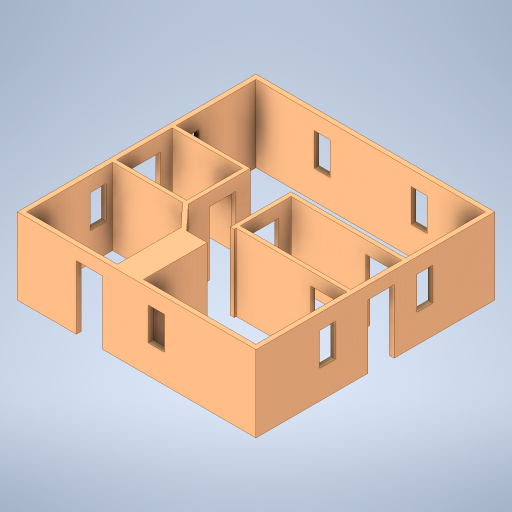
# Autodesk Inventor part: Existing_Kitchen_And_Dining_Room
Saved by Autodesk Inventor 2024 (Build 280153000, 153)
## iProperties
Created: 2023-04-15
Part Number: Existing_Kitchen_And_Dining_Room
Material: Generic
Document SubType Name: Modeling
Designer: Tom
Density: 1 g/cm^3
Appearance: Cherry - Natural Low Gloss
Author: Tom
Autodesk Inventor part; units mm, degrees
ref_plane "YZ Plane" through (0, 0, 0) normal (1, 0, 0) x (0, 1, 0)
ref_plane "XZ Plane" through (0, 0, 0) normal (0, 1, 0) x (-1, 0, 0)
ref_plane "XY Plane" through (0, 0, 0) normal (0, 0, 1) x (1, 0, 0)
sketch "Sketch1" plane through (0, 0, 0) normal (0, 1, 0) x (-1, 0, 0)
  line L0 (149.225, -7470.775) -> (149.225, 149.225)
  line L1 (149.225, 149.225) -> (-7470.775, 149.225)
  line L2 (-7470.775, 149.225) -> (-7470.775, -7470.775)
  line L3 (-7470.775, -7470.775) -> (149.225, -7470.775)
  line L4 (149.225, -2876.55) -> (149.225, -3028.95)
  line L5 (0, 0) -> (0, -7321.55)
  line L6 (0, -7321.55) -> (-7321.55, -7321.55)
  line L7 (-7321.55, -7321.55) -> (-7321.55, 0)
  line L8 (-7321.55, 0) -> (0, 0)
  line L9 (0, -2743.2) -> (-2235.2, -2743.2)
  line L10 (-2235.2, -2743.2) -> (-2895.6, -2032)
  line L11 (-2895.6, -2032) -> (-2895.6, 0)
  line L12 (0, -2873.375) -> (-2235.2, -2873.375)
  line L13 (-2235.2, -2873.375) -> (-2235.2, -4645.3435)
  line L14 (-2235.2, -4645.3435) -> (0, -4645.3435)
  line L15 (0, -4775.5185) -> (-2365.375, -4775.5185)
  line L16 (-2365.375, -4775.5185) -> (-2365.375, -2794.3185)
  line L17 (-2365.375, -2794.3185) -> (-3073.2421, -2032)
  line L18 (-3073.2421, -2032) -> (-3733.6421, -2032)
  line L19 (-3733.6421, -2032) -> (-3733.6421, 0)
  line L20 (-7321.55, -3025.775) -> (-3794.125, -3025.775)
  line L21 (-3794.125, -3025.775) -> (-3794.125, -4645.3435)
  line L22 (-3663.95, -4775.5185) -> (-3663.95, -2832.1)
  line L23 (-3794.125, -2895.6) -> (-7321.55, -2895.6)
  line L24 (-3663.95, -4775.5185) -> (-7321.55, -4775.5185)
  line L25 (-7321.55, -4645.3435) -> (-3794.125, -4645.3435)
  line L26 (-3794.125, -2895.6) -> (-3794.125, -2832.1)
  line L27 (-3794.125, -2832.1) -> (-3663.95, -2832.1)
  dimension "d34" = 7620
  dimension "d37" = 149.225
  dimension "d38" = 7620
  dimension "d39" = 2743.2
  dimension "d40" = 2032
  dimension "d42" = 2235.2
  dimension "d44" = 130.175
  dimension "d47" = 130.175
  dimension "d48" = 1981.2
  dimension "d49" = 130.175
  dimension "d50" = 130.175
  dimension "d52" = 2032
  dimension "d53" = 2895.6
  dimension "d57" = 2895.6
  dimension "d58" = 130.175
  dimension "d62" = 660.4
  dimension "d142" = 130.175
  dimension "d143" = 63.5
  dimension "d144" = 3657.6
  constraints: 56 end point, 12 perpendicular, 10 point on line, 6 horizontal, 4 collinear, 3 parallel, 1 coincident, 3 other
  measures "d34" distance of L1.end L2.end
  measures "d37" distance between parallel lines of L0 L5
  measures "d38" distance of L2.end L0.start
  measures "d39" distance between parallel lines of L8 L9
  measures "d40" distance of L10.end L11.end
  measures "d42" distance of L12.start L12.end
  measures "d44" distance between parallel lines of L9 L12
  measures "d47" distance between parallel lines of L13 L16
  measures "d48" distance of L15.end L16.end
  measures "d49" distance between parallel lines of L15 L14
  measures "d50" distance between parallel lines of L10 L17
  measures "d52" distance of L18.end L19.end
  measures "d53" distance between parallel lines of L5 L11
  measures "d57" distance between parallel lines of L8 L23
  measures "d58" distance between parallel lines of L20 L23
  measures "d62" distance of L17.end L18.end
  measures "d142" distance between parallel lines of L21 L22
  measures "d143" distance between parallel lines of L27 L23
  measures "d144" distance between parallel lines of L7 L22
extrude "Extrusion1" add sketch "Sketch1" along normal blind 2438.4 contours L3 L2 L1 L0 | L5 L12 L13 L14 L15 L16 L17 L18 L19 L8 L11 L10 L9 | L23 L26 L27 L22 L24 L7 L25 L21 L20
sketch "Sketch2" plane through (-149.225, 0, -7470.775) normal (-1, 0, 0) x (0, 0, 1)
  line L0 (4937.125, 1955.8) -> (5445.125, 1955.8)
  line L1 (5445.125, 1955.8) -> (5445.125, 914.4)
  line L2 (5445.125, 914.4) -> (4937.125, 914.4)
  line L3 (4937.125, 914.4) -> (4937.125, 1955.8)
  line L4 (0, 0) -> (7620, 0) projected
  line L5 (2485.7065, 1955.8) -> (1977.7065, 1955.8)
  line L6 (1977.7065, 1955.8) -> (1977.7065, 914.4)
  line L7 (1977.7065, 914.4) -> (2485.7065, 914.4)
  line L8 (2485.7065, 914.4) -> (2485.7065, 1955.8)
  line L9 (3193.7315, 1955.8) -> (4235.1315, 1955.8)
  line L10 (4235.1315, 1955.8) -> (4235.1315, 914.4)
  line L11 (4235.1315, 914.4) -> (3193.7315, 914.4)
  line L12 (3193.7315, 914.4) -> (3193.7315, 1955.8)
  point P0 (7470.775, 0)
  point P1 (4727.575, 2438.4)
  point P2 (2695.2565, 2438.4)
  point P3 (2825.4315, 2438.4)
  dimension "d63" = 914.4
  dimension "d64" = 209.55
  dimension "d65" = 508
  dimension "d66" = 1041.4
  dimension "d67" = 209.55
  dimension "d68" = 508
  dimension "d69" = 1041.4
  dimension "d70" = 914.4
  dimension "d71" = 914.4
  dimension "d72" = 1041.4
  dimension "d73" = 1041.4
  dimension "d74" = 368.3
  constraints: 24 end point, 6 parallel, 3 horizontal, 3 perpendicular
  measures "d63" distance between parallel lines of L4 L2
  measures "d64" distance from line of L3 point (4727.575, 2438.4)
  measures "d65" distance of L0.start L0.end
  measures "d66" distance of L0.end L1.end
  measures "d67" distance from line of L8 point (2695.257, 2438.4)
  measures "d68" distance of L5.start L5.end
  measures "d69" distance of L5.end L6.end
  measures "d70" distance between parallel lines of L4 L7
  measures "d71" distance between parallel lines of L4 L11
  measures "d72" distance of L11.end L9.start
  measures "d73" distance of L9.start L9.end
  measures "d74" distance from line of L12 point (2825.432, 2438.4)
extrude "Extrusion2" cut sketch "Sketch2" against normal up to surface (149.225 mm away)
sketch "Sketch3" plane through (7470.775, 0, -7470.775) normal (0, 0, -1) x (-1, 0, 0)
  line L0 (5105.4, 1955.8) -> (5613.4, 1955.8)
  line L1 (5613.4, 1955.8) -> (5613.4, 914.4)
  line L2 (5613.4, 914.4) -> (5105.4, 914.4)
  line L3 (5105.4, 914.4) -> (5105.4, 1955.8)
  line L4 (0, 0) -> (7620, 0) projected
  line L5 (7470.775, 0) -> (7470.775, 2438.4) projected
  line L6 (2006.6, 1955.8) -> (2514.6, 1955.8)
  line L7 (2514.6, 1955.8) -> (2514.6, 914.4)
  line L8 (2514.6, 914.4) -> (2006.6, 914.4)
  line L9 (2006.6, 914.4) -> (2006.6, 1955.8)
  line L10 (149.225, 0) -> (149.225, 2438.4) projected
  dimension "d78" = 1041.4
  dimension "d79" = 508
  dimension "d80" = 2365.375
  dimension "d81" = 2365.375
  dimension "d82" = 1041.4
  dimension "d83" = 508
  dimension "d84" = 914.4
  dimension "d85" = 914.4
  constraints: 16 end point, 4 parallel, 2 horizontal, 2 perpendicular
  measures "d78" distance of L0.end L1.end
  measures "d79" distance of L0.start L0.end
  measures "d80" distance between parallel lines of L5 L3
  measures "d81" distance between parallel lines of L10 L7
  measures "d82" distance of L6.end L7.end
  measures "d83" distance of L6.start L6.end
  measures "d84" distance between parallel lines of L4 L8
  measures "d85" distance between parallel lines of L4 L2
extrude "Extrusion3" cut sketch "Sketch3" against normal up to surface (149.225 mm away)
sketch "Sketch4" plane through (7470.775, 0, 149.225) normal (1, 0, 0) x (0, 0, -1)
  line L0 (5134.2935, 1955.8) -> (5642.2935, 1955.8)
  line L1 (5642.2935, 1955.8) -> (5642.2935, 914.4)
  line L2 (5642.2935, 914.4) -> (5134.2935, 914.4)
  line L3 (5134.2935, 914.4) -> (5134.2935, 1955.8)
  line L4 (0, 0) -> (7620, 0) projected
  line L5 (2533.65, 1955.8) -> (2025.65, 1955.8)
  line L6 (2025.65, 1955.8) -> (2025.65, 914.4)
  line L7 (2025.65, 914.4) -> (2533.65, 914.4)
  line L8 (2533.65, 914.4) -> (2533.65, 1955.8)
  line L9 (0, 0) -> (0, 2438.4) projected
  line L10 (4794.5685, 0) -> (3175, 0) projected
  line L11 (4410.2347, 0) -> (3572.0347, 0)
  line L12 (3572.0347, 0) -> (3572.0347, 2032)
  line L13 (3572.0347, 2032) -> (4410.2347, 2032)
  line L14 (4410.2347, 2032) -> (4410.2347, 0)
  point P0 (149.225, 0)
  point P1 (4924.7435, 2438.4)
  point P2 (4794.5685, 2438.4)
  dimension "d88" = 209.55
  dimension "d89" = 508
  dimension "d90" = 1041.4
  dimension "d91" = 914.4
  dimension "d92" = 508
  dimension "d94" = 1041.4
  dimension "d97" = 2533.65
  dimension "d98" = 914.4
  dimension "d110" = 838.2
  dimension "d112" = 384.3338
  dimension "d113" = 2032
  constraints: 24 end point, 6 parallel, 3 horizontal, 3 perpendicular, 1 point on line
  measures "d88" distance from line of point (4924.743, 2438.4) L3
  measures "d89" distance of L0.start L0.end
  measures "d90" distance of L0.end L1.end
  measures "d91" distance between parallel lines of L4 L2
  measures "d92" distance of L5.start L5.end
  measures "d94" distance of L7.end L5.start
  measures "d97" distance between parallel lines of L9 L8
  measures "d98" distance between parallel lines of L4 L7
  measures "d110" distance of L12.end L13.end
  measures "d112" distance from line of point (4794.568, 2438.4) L14
  measures "d113" distance of L11.end L12.end
extrude "Extrusion4" cut sketch "Sketch4" against normal up to surface (149.225 mm away)
sketch "Sketch5" plane through (-149.225, 0, 149.225) normal (0, 0, 1) x (1, 0, 0)
  line L0 (0, 0) -> (7620, 0) projected
  line L1 (2724.15, 0) -> (1885.95, 0)
  line L2 (1885.95, 0) -> (1885.95, 2032)
  line L3 (1885.95, 2032) -> (2724.15, 2032)
  line L4 (2724.15, 2032) -> (2724.15, 0)
  line L5 (0, 0) -> (0, 2438.4) projected
  line L6 (4187.6671, 1955.8) -> (4695.6671, 1955.8)
  line L7 (4695.6671, 1955.8) -> (4695.6671, 914.4)
  line L8 (4695.6671, 914.4) -> (4187.6671, 914.4)
  line L9 (4187.6671, 914.4) -> (4187.6671, 1955.8)
  point P0 (149.225, 0)
  point P1 (3882.8671, 2438.4)
  point P2 (1885.95, 0)
  point P3 (149.225, 2438.4)
  dimension "d102" = 838.2
  dimension "d103" = 2032
  dimension "d104" = 304.8
  dimension "d105" = 508
  dimension "d106" = 914.4
  dimension "d107" = 1041.4
  dimension "d114" = 1736.725
  constraints: 16 end point, 4 parallel, 2 horizontal, 2 perpendicular, 1 point on line
  measures "d102" distance between parallel lines of L4 L2
  measures "d103" distance between parallel lines of L0 L3
  measures "d104" distance from line of point (3882.867, 2438.4) L9
  measures "d105" distance of L6.start L6.end
  measures "d106" distance between parallel lines of L0 L8
  measures "d107" distance of L6.end L7.end
  measures "d114" distance from line of L2 point (149.225, 2438.4)
extrude "Extrusion5" cut sketch "Sketch5" against normal up to surface (149.225 mm away)
sketch "Sketch6" plane through (2895.6, 0, -2032) normal (-0.7327935, 0, 0.6804511) x (0.6804511, 0, 0.7327935)
  line L0 (120.8768, 0) -> (-919.4142, 0) projected
  line L1 (-56.1326, 0) -> (-894.3326, 0)
  line L2 (-894.3326, 0) -> (-894.3326, 2032)
  line L3 (-894.3326, 2032) -> (-56.1326, 2032)
  line L4 (-56.1326, 2032) -> (-56.1326, 0)
  line L5 (-970.5326, 0) -> (-970.5326, 2438.4) projected
  point P0 (-481.2778, 0)
  point P1 (-894.3326, 0)
  dimension "d115" = 838.2
  dimension "d116" = 76.2
  dimension "d117" = 2032
  constraints: 8 end point, 2 parallel, 1 horizontal, 1 perpendicular, 1 point on line
  measures "d115" distance of L2.end L3.end
  measures "d116" distance between parallel lines of L5 L2
  measures "d117" distance of L3.end L1.start
extrude "Extrusion6" cut sketch "Sketch6" against normal up to surface (130.175 mm away)
sketch "Sketch7" plane through (2365.375, 0, -2794.3185) normal (1, 0, 0) x (0, 0, -1)
  line L0 (1514.3163, 0) -> (676.1162, 0)
  line L1 (676.1162, 0) -> (676.1162, 2032)
  line L2 (676.1162, 2032) -> (1514.3162, 2032)
  line L3 (1514.3162, 2032) -> (1514.3163, 0)
  line L4 (0, 0) -> (1981.2, 0) projected
  line L5 (1981.2, 0) -> (1981.2, 2438.4) projected
  point P0 (-2794.3185, 0)
  dimension "d120" = 838.2
  dimension "d121" = 466.8838
  dimension "d122" = 2032
  constraints: 8 end point, 2 parallel, 1 collinear, 1 horizontal, 1 perpendicular
  measures "d120" distance of L1.end L2.end
  measures "d121" distance between parallel lines of L5 L3
  measures "d122" distance of L2.end L0.start
extrude "Extrusion7" cut sketch "Sketch7" against normal up to surface (130.175 mm away)
sketch "Sketch8" plane through (3794.125, 0, -3025.775) normal (1, 0, 0) x (0, 0, -1)
  line L0 (1749.7435, 0) -> (-193.675, 0) projected
  line L1 (1228.8837, 0) -> (390.6837, 0)
  line L2 (390.6837, 0) -> (390.6837, 2032)
  line L3 (390.6837, 2032) -> (1228.8837, 2032)
  line L4 (1228.8837, 2032) -> (1228.8837, 0)
  point P0 (-3025.775, 0)
  point P1 (0, 2438.4)
  point P2 (390.6837, 0)
  dimension "d125" = 838.2
  dimension "d126" = 390.6837
  dimension "d127" = 2032
  constraints: 8 end point, 2 parallel, 1 horizontal, 1 perpendicular, 1 point on line
  measures "d125" distance of L2.end L3.end
  measures "d126" distance from line of point (0, 2438.4) L2
  measures "d127" distance of L3.end L1.start
extrude "Extrusion8" cut sketch "Sketch8" against normal up to surface (130.175 mm away)
sketch "Sketch9" plane through (3663.95, 0, -2895.6) normal (0, 0, 1) x (1, 0, 0)
  line L0 (0, 0) -> (3657.6, 0) projected
  line L1 (3352.8, 0) -> (2514.6, 0)
  line L2 (2514.6, 0) -> (2514.6, 2032)
  line L3 (2514.6, 2032) -> (3352.8, 2032)
  line L4 (3352.8, 2032) -> (3352.8, 0)
  point P0 (-3663.95, 0)
  point P1 (3657.6, 2438.4)
  point P2 (2514.6, 0)
  dimension "d130" = 304.8
  dimension "d132" = 2032
  dimension "d133" = 838.2
  constraints: 8 end point, 2 parallel, 1 horizontal, 1 perpendicular, 1 point on line
  measures "d130" distance from line of point (3657.6, 2438.4) L4
  measures "d132" distance of L1.end L2.end
  measures "d133" distance between parallel lines of L2 L4
extrude "Extrusion9" cut sketch "Sketch9" against normal up to surface (130.175 mm away)
sketch "Sketch10" plane through (7321.55, 0, -4775.5185) normal (0, 0, -1) x (-1, 0, 0)
  line L0 (0, 0) -> (3657.6, 0) projected
  line L1 (304.8, 0) -> (1143, 0)
  line L2 (1143, 0) -> (1143, 2032)
  line L3 (1143, 2032) -> (304.8, 2032)
  line L4 (304.8, 2032) -> (304.8, 0)
  point P0 (7321.55, 0)
  point P1 (0, 2438.4)
  point P2 (1143, 0)
  dimension "d136" = 2032
  dimension "d137" = 304.8
  dimension "d138" = 838.2
  constraints: 8 end point, 2 parallel, 1 horizontal, 1 perpendicular, 1 point on line
  measures "d136" distance of L1.end L2.end
  measures "d137" distance from line of point (0, 2438.4) L4
  measures "d138" distance of L2.end L3.end
extrude "Extrusion10" cut sketch "Sketch10" against normal up to surface (130.175 mm away)
body "Solid1"
